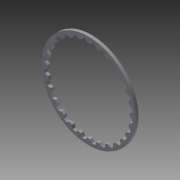
# Autodesk Inventor part: Ring
Saved by Autodesk Inventor 2013 (Build 170138000, 138)
## iProperties
Created: 2014-02-12
Part Number: Ring
Material: Generic
Document SubType Name: Modeling
Designer: robotics
Density: 1 g/cm^3
Author: robotics
Autodesk Inventor part; units mm, degrees
ref_plane "YZ Plane" through (0, 0, 0) normal (1, 0, 0) x (0, 1, 0)
ref_plane "XZ Plane" through (0, 0, 0) normal (0, 1, 0) x (-1, 0, 0)
ref_plane "XY Plane" through (0, 0, 0) normal (0, 0, 1) x (1, 0, 0)
sketch "Sketch1" plane through (0, 0, 0) normal (0, 0, 1) x (1, 0, 0)
  line L0 (0, 0) -> (0, 8.6937) construction
  line L1 (1.8646, 23.6385) -> (0.7937, 22.1875)
  line L2 (0.7937, 22.1875) -> (0, 22.1875)
  line L3 (-1.8646, 23.6385) -> (-0.7937, 22.1875)
  line L4 (-0.7937, 22.1875) -> (0, 22.1875)
  line L5 (-0.7937, 22.1875) -> (0.7937, 22.1875)
  line L6 (-3.4422, 23.4607) -> (-4.1633, 21.8078)
  line L7 (-4.1633, 21.8078) -> (-4.9372, 21.6312)
  line L8 (-7.078, 22.6309) -> (-5.711, 21.4546)
  line L9 (-5.711, 21.4546) -> (-4.9372, 21.6312)
  line L10 (-8.5764, 22.1066) -> (-8.9116, 20.3346)
  line L11 (-8.9116, 20.3346) -> (-9.6268, 19.9902)
  line L12 (-11.9363, 20.4885) -> (-10.3419, 19.6458)
  line L13 (-10.3419, 19.6458) -> (-9.6268, 19.9902)
  line L14 (-13.2805, 19.6439) -> (-13.2131, 17.8418)
  line L15 (-13.2131, 17.8418) -> (-13.8337, 17.3469)
  line L16 (-16.1962, 17.3187) -> (-14.4542, 16.852)
  line L17 (-14.4542, 16.852) -> (-13.8337, 17.3469)
  line L18 (-17.3187, 16.1962) -> (-16.852, 14.4542)
  line L19 (-16.852, 14.4542) -> (-17.3469, 13.8337)
  line L20 (-19.6439, 13.2805) -> (-17.8418, 13.2131)
  line L21 (-17.8418, 13.2131) -> (-17.3469, 13.8337)
  line L22 (-20.4885, 11.9363) -> (-19.6458, 10.3419)
  line L23 (-19.6458, 10.3419) -> (-19.9902, 9.6268)
  line L24 (-22.1066, 8.5764) -> (-20.3346, 8.9116)
  line L25 (-20.3346, 8.9116) -> (-19.9902, 9.6268)
  line L26 (-22.6309, 7.078) -> (-21.4546, 5.711)
  line L27 (-21.4546, 5.711) -> (-21.6312, 4.9372)
  line L28 (-23.4607, 3.4422) -> (-21.8078, 4.1633)
  line L29 (-21.8078, 4.1633) -> (-21.6312, 4.9372)
  line L30 (-23.6385, 1.8646) -> (-22.1875, 0.7937)
  line L31 (-22.1875, 0.7937) -> (-22.1875, 0)
  line L32 (-23.6385, -1.8646) -> (-22.1875, -0.7937)
  line L33 (-22.1875, -0.7937) -> (-22.1875, 0)
  line L34 (-23.4607, -3.4422) -> (-21.8078, -4.1633)
  line L35 (-21.8078, -4.1633) -> (-21.6312, -4.9372)
  line L36 (-22.6309, -7.078) -> (-21.4546, -5.711)
  line L37 (-21.4546, -5.711) -> (-21.6312, -4.9372)
  line L38 (-22.1066, -8.5764) -> (-20.3346, -8.9116)
  line L39 (-20.3346, -8.9116) -> (-19.9902, -9.6268)
  line L40 (-20.4885, -11.9363) -> (-19.6458, -10.3419)
  line L41 (-19.6458, -10.3419) -> (-19.9902, -9.6268)
  line L42 (-19.6439, -13.2805) -> (-17.8418, -13.2131)
  line L43 (-17.8418, -13.2131) -> (-17.3469, -13.8337)
  line L44 (-17.3187, -16.1962) -> (-16.852, -14.4542)
  line L45 (-16.852, -14.4542) -> (-17.3469, -13.8337)
  line L46 (-16.1962, -17.3187) -> (-14.4542, -16.852)
  line L47 (-14.4542, -16.852) -> (-13.8337, -17.3469)
  line L48 (-13.2805, -19.6439) -> (-13.2131, -17.8418)
  line L49 (-13.2131, -17.8418) -> (-13.8337, -17.3469)
  line L50 (-11.9363, -20.4885) -> (-10.3419, -19.6458)
  line L51 (-10.3419, -19.6458) -> (-9.6268, -19.9902)
  line L52 (-8.5764, -22.1066) -> (-8.9116, -20.3346)
  line L53 (-8.9116, -20.3346) -> (-9.6268, -19.9902)
  line L54 (-7.078, -22.6309) -> (-5.711, -21.4546)
  line L55 (-5.711, -21.4546) -> (-4.9372, -21.6312)
  line L56 (-3.4422, -23.4607) -> (-4.1633, -21.8078)
  line L57 (-4.1633, -21.8078) -> (-4.9372, -21.6312)
  line L58 (-1.8646, -23.6385) -> (-0.7938, -22.1875)
  line L59 (-0.7938, -22.1875) -> (0, -22.1875)
  line L60 (1.8646, -23.6385) -> (0.7937, -22.1875)
  line L61 (0.7937, -22.1875) -> (0, -22.1875)
  line L62 (3.4422, -23.4607) -> (4.1633, -21.8078)
  line L63 (4.1633, -21.8078) -> (4.9372, -21.6312)
  line L64 (7.078, -22.6309) -> (5.711, -21.4546)
  line L65 (5.711, -21.4546) -> (4.9372, -21.6312)
  line L66 (8.5764, -22.1066) -> (8.9116, -20.3346)
  line L67 (8.9116, -20.3346) -> (9.6268, -19.9902)
  line L68 (11.9363, -20.4885) -> (10.3419, -19.6458)
  line L69 (10.3419, -19.6458) -> (9.6268, -19.9902)
  line L70 (13.2805, -19.6439) -> (13.2131, -17.8418)
  line L71 (13.2131, -17.8418) -> (13.8337, -17.3469)
  line L72 (16.1962, -17.3187) -> (14.4542, -16.852)
  line L73 (14.4542, -16.852) -> (13.8337, -17.3469)
  line L74 (17.3187, -16.1962) -> (16.852, -14.4542)
  line L75 (16.852, -14.4542) -> (17.3469, -13.8337)
  line L76 (19.6439, -13.2805) -> (17.8418, -13.2131)
  line L77 (17.8418, -13.2131) -> (17.3469, -13.8337)
  line L78 (20.4885, -11.9363) -> (19.6458, -10.3419)
  line L79 (19.6458, -10.3419) -> (19.9902, -9.6268)
  line L80 (22.1066, -8.5764) -> (20.3346, -8.9116)
  line L81 (20.3346, -8.9116) -> (19.9902, -9.6268)
  line L82 (22.6309, -7.078) -> (21.4546, -5.711)
  line L83 (21.4546, -5.711) -> (21.6312, -4.9372)
  line L84 (23.4607, -3.4422) -> (21.8078, -4.1633)
  line L85 (21.8078, -4.1633) -> (21.6312, -4.9372)
  line L86 (23.6385, -1.8646) -> (22.1875, -0.7938)
  line L87 (22.1875, -0.7938) -> (22.1875, 0)
  line L88 (23.6385, 1.8646) -> (22.1875, 0.7938)
  line L89 (22.1875, 0.7938) -> (22.1875, 0)
  line L90 (23.4607, 3.4422) -> (21.8078, 4.1633)
  line L91 (21.8078, 4.1633) -> (21.6312, 4.9372)
  line L92 (22.6309, 7.078) -> (21.4546, 5.711)
  line L93 (21.4546, 5.711) -> (21.6312, 4.9372)
  line L94 (22.1066, 8.5764) -> (20.3346, 8.9116)
  line L95 (20.3346, 8.9116) -> (19.9902, 9.6268)
  line L96 (20.4885, 11.9363) -> (19.6458, 10.3419)
  line L97 (19.6458, 10.3419) -> (19.9902, 9.6268)
  line L98 (19.6439, 13.2805) -> (17.8418, 13.2131)
  line L99 (17.8418, 13.2131) -> (17.3469, 13.8337)
  line L100 (17.3187, 16.1962) -> (16.852, 14.4542)
  line L101 (16.852, 14.4542) -> (17.3469, 13.8337)
  line L102 (16.1962, 17.3187) -> (14.4542, 16.852)
  line L103 (14.4542, 16.852) -> (13.8337, 17.3469)
  line L104 (13.2805, 19.6439) -> (13.2131, 17.8418)
  line L105 (13.2131, 17.8418) -> (13.8337, 17.3469)
  line L106 (11.9363, 20.4885) -> (10.3419, 19.6458)
  line L107 (10.3419, 19.6458) -> (9.6268, 19.9902)
  line L108 (8.5764, 22.1066) -> (8.9116, 20.3346)
  line L109 (8.9116, 20.3346) -> (9.6268, 19.9902)
  line L110 (7.078, 22.6309) -> (5.711, 21.4546)
  line L111 (5.711, 21.4546) -> (4.9372, 21.6312)
  line L112 (3.4422, 23.4607) -> (4.1633, 21.8078)
  line L113 (4.1633, 21.8078) -> (4.9372, 21.6312)
  line L114 (-3.4422, 23.4607) -> (-1.8646, 23.6385) construction
  circle A0 centre (0, 0) radius 25.2994
  arc A1 (-11.9363, 20.4885) -> (-13.2805, 19.6439) centre (0, 0) ccw
  arc A2 (-7.078, 22.6309) -> (-8.5764, 22.1066) centre (0, 0) ccw
  arc A3 (-1.8646, 23.6385) -> (-3.4422, 23.4607) centre (0, 0) ccw
  arc A4 (3.4422, 23.4607) -> (1.8646, 23.6385) centre (0, 0) ccw
  arc A5 (8.5764, 22.1066) -> (7.078, 22.6309) centre (0, 0) ccw
  arc A6 (13.2805, 19.6439) -> (11.9363, 20.4885) centre (0, 0) ccw
  arc A7 (17.3187, 16.1962) -> (16.1962, 17.3187) centre (0, 0) ccw
  arc A8 (20.4885, 11.9363) -> (19.6439, 13.2805) centre (0, 0) ccw
  arc A9 (22.6309, 7.078) -> (22.1066, 8.5764) centre (0, 0) ccw
  arc A10 (23.6385, 1.8646) -> (23.4607, 3.4422) centre (0, 0) ccw
  arc A11 (23.4607, -3.4422) -> (23.6385, -1.8646) centre (0, 0) ccw
  arc A12 (22.1066, -8.5764) -> (22.6309, -7.078) centre (0, 0) ccw
  arc A13 (19.6439, -13.2805) -> (20.4885, -11.9363) centre (0, 0) ccw
  arc A14 (16.1962, -17.3187) -> (17.3187, -16.1962) centre (0, 0) ccw
  arc A15 (11.9363, -20.4885) -> (13.2805, -19.6439) centre (0, 0) ccw
  arc A16 (7.078, -22.6309) -> (8.5764, -22.1066) centre (0, 0) ccw
  arc A17 (1.8646, -23.6385) -> (3.4422, -23.4607) centre (0, 0) ccw
  arc A18 (-3.4422, -23.4607) -> (-1.8646, -23.6385) centre (0, 0) ccw
  arc A19 (-8.5764, -22.1066) -> (-7.078, -22.6309) centre (0, 0) ccw
  arc A20 (-13.2805, -19.6439) -> (-11.9363, -20.4885) centre (0, 0) ccw
  arc A21 (-17.3187, -16.1962) -> (-16.1962, -17.3187) centre (0, 0) ccw
  arc A22 (-20.4885, -11.9363) -> (-19.6439, -13.2805) centre (0, 0) ccw
  arc A23 (-22.6309, -7.078) -> (-22.1066, -8.5764) centre (0, 0) ccw
  arc A24 (-23.6385, -1.8646) -> (-23.4607, -3.4422) centre (0, 0) ccw
  arc A25 (-23.4607, 3.4422) -> (-23.6385, 1.8646) centre (0, 0) ccw
  arc A26 (-22.1066, 8.5764) -> (-22.6309, 7.078) centre (0, 0) ccw
  arc A27 (-16.1962, 17.3187) -> (-17.3187, 16.1962) centre (0, 0) ccw
  arc A28 (-19.6439, 13.2805) -> (-20.4885, 11.9363) centre (0, 0) ccw
  dimension "d0" = 1.5875
  dimension "d2" = 1.8034
  dimension "d5" = 360
  dimension "d7" = 120
  dimension "d9" = 1.5875
  constraints: 230 end point, 56 point on circle, 29 centre point, 3 coincident, 2 symmetric about line, 1 collinear, 1 equal length, 1 perpendicular, 1 point on line, 1 vertical, 253 other
  measures "d0" distance of L3.end L1.end
  measures "d2" distance of L1.start L1.end
  measures "d7" angle of L3 L114
  measures "d9" radial gap between concentric circles of A2 A0
extrude "Extrusion1" add sketch "Sketch1" along normal blind 1.5875
body "Solid1"
